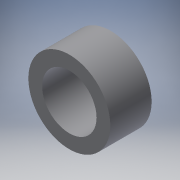
# Autodesk Inventor part: Wheel_Tire
Saved by Autodesk Inventor 2019 (Build 230136000, 136)
## iProperties
Created: 2019-03-02
Part Number: Wheel_Tire
Material: Generic
Document SubType Name: Modeling
Designer: alarr
Density: 1 g/cm^3
Appearance: Default
Author: alarr
Autodesk Inventor part; units mm, degrees
ref_plane "YZ Plane" through (0, 0, 0) normal (1, 0, 0) x (0, 1, 0)
ref_plane "XZ Plane" through (0, 0, 0) normal (0, 1, 0) x (-1, 0, 0)
ref_plane "XY Plane" through (0, 0, 0) normal (0, 0, 1) x (1, 0, 0)
sketch "Sketch1" plane through (0, 0, 0) normal (0, 0, 1) x (1, 0, 0)
  circle A0 centre (0, 0) radius 50.165 projected
  circle A1 centre (0, 0) radius 50.165
  circle A2 centre (0, 0) radius 75.565
  point P0 (0, 0)
  dimension "d0" = 25.4
  constraints: 2 centre point, 1 coincident, 1 concentric
  measures "d0" radial gap between concentric circles of A0 A2
extrude "Extrusion1" add sketch "Sketch1" along normal mid plane 82.55
body "Solid1"
